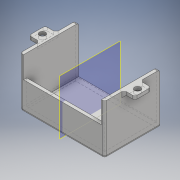
# Autodesk Inventor part: Eletronica - protecaoFonte
Saved by Autodesk Inventor 2017 (Build 210142000, 142)
## iProperties
Created: 2020-10-24
Part Number: Eletronica - protecaoFonte
Material: Generic
Document SubType Name: Modeling
Designer: ale
Density: 1 g/cm^3
Appearance: Default
Author: ale
Autodesk Inventor part; units mm, degrees
ref_plane "YZ Plane" through (0, 0, 0) normal (1, 0, 0) x (0, 1, 0)
ref_plane "XZ Plane" through (0, 0, 0) normal (0, 1, 0) x (-1, 0, 0)
ref_plane "XY Plane" through (0, 0, 0) normal (0, 0, 1) x (1, 0, 0)
sketch "Sketch1" plane through (0, 0, 0) normal (0, 0, 1) x (1, 0, 0)
  line L0 (-36, 22.5) -> (36, 22.5)
  line L1 (36, 22.5) -> (36, -22.5)
  line L2 (36, -22.5) -> (-36, -22.5)
  line L3 (-36, -22.5) -> (-36, 22.5)
  line L4 (-36, 22.5) -> (36, -22.5) construction
  line L5 (36, 22.5) -> (-36, -22.5) construction
  line L6 (39, 25.5) -> (-39, 25.5)
  line L7 (-39, 25.5) -> (-39, -25.5)
  line L8 (-39, -25.5) -> (39, -25.5)
  line L9 (39, -25.5) -> (39, 25.5)
  point P0 (0, 0)
  dimension "d0" = 72
  dimension "d1" = 45
  dimension "d2" = 3
  constraints: 20 end point, 4 parallel, 2 midpoint, 2 perpendicular, 1 horizontal, 3 other
  measures "d0" distance of L1.end L2.end
  measures "d1" distance of L0.end L1.end
  measures "d2" distance between parallel lines of L0 L6
extrude "Extrusion1" add sketch "Sketch1" along normal blind 43
sketch "Sketch2" plane through (0, 0, 0) normal (0, 0, -1) x (-1, 0, 0)
  line L0 (-39, 25.5) -> (39, 25.5) projected
  line L1 (39, 25.5) -> (39, -25.5) projected
  line L2 (-39, 25.5) -> (39, 25.5)
  line L3 (39, 25.5) -> (39, -25.5)
  line L4 (39, -25.5) -> (-39, -25.5)
  line L5 (-39, -25.5) -> (-39, 25.5)
  point P0 (0, 0)
  constraints: 8 end point, 2 parallel, 1 horizontal, 1 perpendicular
extrude "Extrusion2" add sketch "Sketch2" along normal blind 3
sketch "Sketch3" plane through (-39, 25.5, 43) normal (0, 1, 0) x (1, 0, 0)
  line L0 (3, 43) -> (75, 43) projected
  line L1 (75, 43) -> (75, 0) projected
  line L2 (3, 43) -> (75, 43)
  line L3 (75, 43) -> (75, 0)
  line L4 (75, 0) -> (3, 0)
  line L5 (3, 0) -> (3, 43)
  point P0 (39, 43)
  constraints: 8 end point, 2 parallel, 1 horizontal, 1 perpendicular
extrude "Extrusion3" cut sketch "Sketch3" against normal up to surface (3 mm away)
ref_plane "Work Plane1" through (0, -25.5, 43) normal (-1, 0, 0) x (0, 0, 1)
sketch "Sketch5" plane through (0, 0, 43) normal (0, 0, 1) x (1, 0, 0)
  line L0 (-39, -25.5) -> (-39, 25.5) projected
  line L1 (-39, 7.5) -> (-47, 7.5)
  line L2 (-49, 5.5) -> (-49, -5.5)
  line L3 (-47, -7.5) -> (-39, -7.5)
  line L4 (-39, -7.5) -> (-39, 7.5)
  line L5 (-36, 25.5) -> (-39, 25.5) projected
  circle A0 centre (-44, 0) radius 2.75
  arc A1 (-49, -5.5) -> (-47, -7.5) centre (-47, -5.5) ccw
  arc A2 (-47, 7.5) -> (-49, 5.5) centre (-47, 5.5) ccw
  point P0 (0, 0)
  point P1 (-49, -7.5)
  point P2 (-49, 7.5)
  dimension "d12" = 10
  dimension "d13" = 15
  dimension "d14" = 18
  dimension "d17" = 5.5
  dimension "d18" = 5
  dimension "d21" = 2
  constraints: 8 end point, 5 point on line, 4 point on circle, 4 tangent, 3 centre point, 2 parallel, 1 equal radius, 1 horizontal, 1 perpendicular
  measures "d12" distance of L3.end point (-49, -7.5)
  measures "d13" distance of point (-49, -7.5) point (-49, 7.5)
  measures "d14" distance between parallel lines of L5 L1
  measures "d17" diameter of A0
  measures "d18" distance from line of A0.centre L0
  measures "d21" radius of A1
extrude "Extrusion5" add sketch "Sketch5" against normal blind 3
mirror "Mirror1" about plane through (0, -25.5, 43) normal (-1, 0, 0) of "Extrusion5"
chamfer "Chamfer1" distance 2 angle 45 6 edges at (-39, 0, 40) (-39, 7.5, 41.5) (-39, -7.5, 41.5) (39, 0, 40) (39, -7.5, 41.5) (39, 7.5, 41.5)
fillet "Fillet1" radius 2 8 edges at (39, 0, -3) (-39, 0, -3) (-39, -25.5, 20) (0, -25.5, -3) (39, -25.5, 20) (0, 25.5, -3) (-37.5, 25.5, 43) (37.5, 25.5, 43)
sketch "Sketch7" plane through (-37, -25.5, -1) normal (0, -1, 0) x (1, 0, 0)
  line L0 (73, 44) -> (1, 44) projected
  line L1 (1, 1) -> (1, 44) projected
  line L2 (73, 44) -> (1, 44)
  line L3 (1, 44) -> (1, 24)
  line L4 (1, 24) -> (73, 24)
  line L5 (73, 24) -> (73, 44)
  point P0 (37, 1)
  dimension "d26" = 20
  constraints: 8 end point, 2 parallel, 1 horizontal, 1 perpendicular, 1 point on line
  measures "d26" distance between parallel lines of L0 L4
extrude "Extrusion6" cut sketch "Sketch7" against normal up to surface (3 mm away)
equation "\"d18\" = 0.5 * d12"
body "Solid1"
